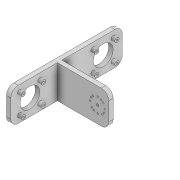
# Autodesk Inventor part: StereoVisionHolder_3
Saved by Autodesk Inventor 2022 (Build 260153000, 153)
## iProperties
Created: 2022-11-13
Part Number: StereoVisionHolder_3
Material: Generic
Document SubType Name: Modeling
Designer: MVeszpremi
Density: 1 g/cm^3
Appearance: Default
Author: MVeszpremi
Autodesk Inventor part; units mm, degrees
ref_plane "YZ Plane" through (0, 0, 0) normal (1, 0, 0) x (0, 1, 0)
ref_plane "XZ Plane" through (0, 0, 0) normal (0, 1, 0) x (-1, 0, 0)
ref_plane "XY Plane" through (0, 0, 0) normal (0, 0, 1) x (1, 0, 0)
sketch "Sketch1" plane through (0, 0, 0) normal (0, 0, 1) x (1, 0, 0)
  line L0 (0, 0) -> (20, 0)
  line L1 (20, 0) -> (20, 35)
  line L2 (20, 35) -> (0, 35)
  line L3 (0, 35) -> (0, 0)
  circle A0 centre (0, 35) radius 1.5
  circle A1 centre (20, 35) radius 1.5
  circle A2 centre (0, 0) radius 1.5
  circle A3 centre (20, 0) radius 1.5
  line L4 (0, 35) -> (20, 0)
  line L5 (-15, -5) -> (20, -5)
  line L6 (20, -5) -> (20, 40)
  line L7 (20, 40) -> (-15, 40)
  line L8 (-15, 40) -> (-15, -5)
  line L9 (20, 40) -> (25, 40)
  line L10 (25, 40) -> (25, -5)
  line L11 (25, -5) -> (20, -5)
  line L12 (20, -5) -> (20, 40)
  point P0 (10, 17.5)
  point P1 (20, 36.5)
  point P2 (20, 33.5)
  point P3 (20, 1.5)
  point P4 (20, -1.5)
  dimension "d0" = 35
  dimension "d1" = 20
  dimension "d2" = 3
  dimension "d3" = 3
  dimension "d4" = 3
  dimension "d5" = 3
  dimension "d6" = 5
  dimension "d7" = 15
  dimension "d45" = 5
  dimension "d46" = 45
  dimension "d47" = 10
  constraints: 26 end point, 6 parallel, 4 centre point, 4 coincident, 3 horizontal, 3 perpendicular, 1 midpoint
  measures "d0" distance of L2.end L0.start
  measures "d1" distance of L1.end L2.end
  measures "d2" diameter of A0
  measures "d3" diameter of A1
  measures "d4" diameter of A2
  measures "d5" diameter of A3
  measures "d6" distance between parallel lines of L2 L7
  measures "d7" distance between parallel lines of L8 L3
  measures "d45" distance of L6.end L9.end
  measures "d46" distance between parallel lines of L11 L9
  measures "d47" distance from line of L6 point (10, 17.5)
extrude "Extrusion1" add sketch "Sketch1" along normal blind 5 contours A2 L3 A0 L4 A3 L0 | L0 A3 L6 L5 L8 L7 A1 L2 A0 L3 A2 | L4 A0 L2 A1 L1 A3 | A3 L1 A1 L6 L9 L10 L11
sketch "Sketch2" plane through (0, 0, 5) normal (0, 0, 1) x (1, 0, 0)
  line L0 (30, 40) -> (-15, 40) projected
  line L1 (-15, 40) -> (-21, 40)
  line L2 (-21, 40) -> (-21, -5)
  line L3 (-21, -5) -> (-15, -5)
  line L4 (-15, -5) -> (-15, 40)
  point P0 (0, 0)
  dimension "d10" = 6
  constraints: 8 end point, 2 parallel, 1 coincident, 1 horizontal, 1 perpendicular
  measures "d10" distance of L0.end L1.end
extrude "Extrusion2" add sketch "Sketch2" along normal blind 147 and the other way blind 5
ref_plane "Work Plane2" through (0, 0, 76) normal (0, 0, -1) x (-1, 0, 0)
mirror "Mirror2" about plane through (0, 0, 76) normal (0, 0, -1) of "Extrusion1"
sketch "Sketch3" plane through (-15, -5, 5) normal (1, 0, 0) x (0, 0, -1)
  line L0 (-142, 45) -> (-142, 0) projected
  line L1 (-142, 22.5) -> (0, 22.5)
  line L2 (0, 45) -> (0, 0) projected
  circle A0 centre (-121, 22.5) radius 13.5
  circle A1 centre (-21, 22.5) radius 13.5
  line L3 (-134.75, 36.25) -> (-107.25, 36.25)
  line L4 (-107.25, 36.25) -> (-107.25, 8.75)
  line L5 (-107.25, 8.75) -> (-134.75, 8.75)
  line L6 (-134.75, 8.75) -> (-134.75, 36.25)
  line L7 (-134.75, 36.25) -> (-107.25, 8.75) construction
  line L8 (-107.25, 36.25) -> (-134.75, 8.75) construction
  line L9 (0, 45) -> (-142, 45) projected
  line L10 (-7.25, 8.75) -> (-34.75, 8.75)
  line L11 (-34.75, 8.75) -> (-34.75, 36.25)
  line L12 (-34.75, 36.25) -> (-7.25, 36.25)
  line L13 (-7.25, 36.25) -> (-7.25, 8.75)
  line L14 (-7.25, 8.75) -> (-34.75, 36.25) construction
  line L15 (-34.75, 8.75) -> (-7.25, 36.25) construction
  circle A2 centre (-134.75, 36.25) radius 3
  circle A3 centre (-107.25, 36.25) radius 3
  circle A4 centre (-107.25, 8.75) radius 3
  circle A5 centre (-134.75, 8.75) radius 3
  circle A6 centre (-34.75, 36.25) radius 3
  circle A7 centre (-7.25, 36.25) radius 3
  circle A8 centre (-7.25, 8.75) radius 3
  circle A9 centre (-34.75, 8.75) radius 3
  circle A10 centre (-134.75, 36.25) radius 1.25
  circle A11 centre (-107.25, 36.25) radius 1.25
  circle A12 centre (-107.25, 8.75) radius 1.25
  circle A13 centre (-134.75, 8.75) radius 1.25
  circle A14 centre (-34.75, 36.25) radius 1.25
  circle A15 centre (-7.25, 36.25) radius 1.25
  circle A16 centre (-34.75, 8.75) radius 1.25
  circle A17 centre (-7.25, 8.75) radius 1.25
  point P0 (5, 5)
  point P1 (-102, 45)
  dimension "d16" = 27
  dimension "d17" = 27
  dimension "d18" = 27.5
  dimension "d19" = 27.5
  dimension "d20" = 22.5
  dimension "d21" = 21
  dimension "d22" = 21
  dimension "d23" = 27.5
  dimension "d24" = 27.5
  dimension "d25" = 6
  dimension "d26" = 6
  dimension "d27" = 6
  dimension "d28" = 6
  dimension "d29" = 6
  dimension "d30" = 6
  dimension "d31" = 6
  dimension "d32" = 6
  dimension "d33" = 2.5
  dimension "d34" = 2.5
  dimension "d35" = 2.5
  dimension "d36" = 2.5
  dimension "d37" = 2.5
  dimension "d38" = 2.5
  dimension "d39" = 2.5
  dimension "d40" = 2.5
  constraints: 26 end point, 18 centre point, 16 coincident, 5 midpoint, 4 parallel, 3 horizontal, 2 perpendicular, 2 point on line, 2 other
  measures "d16" diameter of A0
  measures "d17" diameter of A1
  measures "d18" distance of L4.end L5.end
  measures "d19" distance of L3.end L4.end
  measures "d20" distance between parallel lines of L9 L1
  measures "d22" distance from line of L2 A1.centre
  measures "d23" distance of L11.end L12.end
  measures "d24" distance of L10.end L11.end
  measures "d25" diameter of A3
  measures "d26" diameter of A2
  measures "d27" diameter of A5
  measures "d28" diameter of A4
  measures "d29" diameter of A9
  measures "d30" diameter of A6
  measures "d31" diameter of A7
  measures "d32" diameter of A8
  measures "d33" diameter of A10
  measures "d34" diameter of A11
  measures "d35" diameter of A12
  measures "d36" diameter of A13
  measures "d37" diameter of A14
  measures "d38" diameter of A15
  measures "d39" diameter of A16
  measures "d40" diameter of A17
extrude "Extrusion3" cut sketch "Sketch3" against normal blind 6 contours A0 L1 | L1 A0 | A13 L5 L6 | L6 L5 A13 | A10 L3 L6 | L6 L3 A10 | A1 L1 | L1 A1 | A15 L12 L13 | L13 L12 A15 | A17 L10 L13 | L13 L10 A17 | A12 L4 L5 | L5 L4 A12 | A11 L4 L3 | L3 L4 A11 | A14 L11 L12 | L12 L11 A14 | A16 L11 L10 | L10 L11 A16
extrude "Extrusion4" add sketch "Sketch3" along normal blind 5 contours A5 L5 A13 L6 | L6 A13 L5 A5 | A2 L3 A10 L6 | L6 A10 L3 A2 | A7 L12 A15 L13 | L13 A15 L12 A7 | A8 L10 A17 L13 | L13 A17 L10 A8 | A4 L4 A12 L5 | L5 A12 L4 A4 | A3 L4 A11 L3 | L3 A11 L4 A3 | A6 L11 A14 L12 | L12 A14 L11 A6 | A9 L11 A16 L10 | L10 A16 L11 A9
sketch "Sketch4" plane through (25, -5, 0) normal (1, 0, 0) x (0, 0, -1)
  line L0 (-152, 0) -> (-152, 45) projected
  line L1 (-152, 0) -> (-147, 0) projected
  line L2 (-147, 0) -> (-147, 45) projected
  line L3 (-152, 45) -> (-147, 45) projected
  line L4 (0, 0) -> (0, 45) projected
  line L5 (0, 45) -> (-5, 45) projected
  line L6 (-5, 0) -> (-5, 45) projected
  line L7 (0, 0) -> (-5, 0) projected
  point P0 (0, 5)
extrude "Extrusion5" cut sketch "Sketch4" against normal up to surface (40 mm away)
fillet "Fillet5" radius 10 4 edges at (-18, -5, 152) (-18, 40, 152) (-18, -5, 0) (-18, 40, 0)
sketch "Sketch8" plane through (-15, 5, 152) normal (1, 0, 0) x (0, 0, -1)
  line L0 (10, 35) -> (142, 35) projected
  line L1 (142, -10) -> (10, -10) projected
  line L2 (63.5, 35) -> (69.5, 35)
  line L3 (69.5, 35) -> (69.5, -10)
  line L4 (69.5, -10) -> (63.5, -10)
  line L5 (63.5, -10) -> (63.5, 35)
  line L6 (0, 0) -> (0, 25) projected
  line L7 (76, 35) -> (76, 67.6584)
  point P0 (152, -5)
  dimension "d84" = 6
  dimension "d86" = 12.5
  constraints: 10 end point, 2 parallel, 2 point on line, 1 horizontal, 1 midpoint, 1 perpendicular, 1 vertical
  measures "d84" distance between parallel lines of L5 L3
  measures "d86" distance between parallel lines of L7 L5
extrude "Extrusion10" add sketch "Sketch8" along normal blind 70
fillet "Fillet6" radius 10 2 edges at (55, -5, 85.5) (55, 40, 85.5)
sketch "Sketch9" plane through (-15, -5, 88.5) normal (0, 0, 1) x (1, 0, 0)
  line L0 (70, 22.5) -> (55, 22.5)
  circle A0 centre (55, 22.5) radius 10
  circle A1 centre (65, 22.5) radius 1
  circle A2 centre (55, 32.5) radius 1
  circle A3 centre (45, 22.5) radius 1
  circle A4 centre (55, 12.5) radius 1
  circle A5 centre (63.6603, 17.5) radius 1
  line L1 (55, 22.5) -> (63.6603, 17.5)
  line L2 (55, 22.5) -> (61.4279, 14.8396)
  circle A6 centre (61.4279, 14.8396) radius 1
  circle A7 centre (60, 31.1603) radius 1
  circle A8 centre (62.6604, 28.9279) radius 1
  circle A9 centre (46.3397, 27.5) radius 1
  circle A10 centre (48.5721, 30.1604) radius 1
  circle A11 centre (50, 13.8397) radius 1
  circle A12 centre (47.3396, 16.0721) radius 1
  line L3 (70, 10) -> (70, 35) projected
  line L4 (70, 35) -> (70, 10)
  circle A13 centre (55, 22.5) radius 1.45
  point P0 (15, 5)
  dimension "d94" = 20
  dimension "d96" = 2
  dimension "d97" = 360
  dimension "d98" = 30
  dimension "d99" = 2
  dimension "d100" = 2
  dimension "d101" = 50
  dimension "d102" = 360
  dimension "d103" = 15
  dimension "d104" = 2.9
  constraints: 14 centre point, 8 end point, 3 coincident, 3 point on circle, 1 collinear, 1 horizontal, 1 midpoint, 1 point on line, 26 other
  measures "d94" diameter of A0
  measures "d96" diameter of A1
  measures "d98" angle of L0 L1
  measures "d99" diameter of A5
  measures "d100" diameter of A6
  measures "d101" angle of L0 L2
  measures "d103" distance of L0.start L0.end
  measures "d104" diameter of A13
extrude "Extrusion11" cut sketch "Sketch9" against normal blind 70 contours A1 A0 L0 | L0 A0 A1 | A0 A1 L0 | L0 A1 A0 | A8 A0 | A0 A8 | A5 A0 | A0 L1 A5 | A13 L1 L0 | L0 L2 A13 | A0 A5 L1 | L1 A13 L2 | A7 A0 | A0 A7 | A6 A0 L2 | L2 A0 A6 | A6 A0 | A2 A0 | A0 A2 | A4 A0 | A0 A4 | A10 A0 | A0 A10 | A11 A0 | A0 A11 | A9 A0 | A0 A9 | A12 A0 | A0 A12 | A3 A0 | A0 A3
equation "\"d41\" = d30"
body "Solid1"
